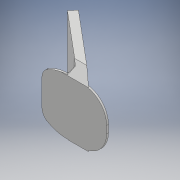
# Autodesk Inventor part: forJ
Saved by Autodesk Inventor 2018 (Build 220112000, 112)
## iProperties
Created: 2019-10-10
Part Number: forJ
Material: Типовые
Document SubType Name: Modeling
Designer: Professional
Density: 1 g/cm^3
Appearance: По умолчанию
Author: Professional
Autodesk Inventor part; units mm, degrees
ref_plane "YZ Plane" through (0, 0, 0) normal (1, 0, 0) x (0, 1, 0)
ref_plane "XZ Plane" through (0, 0, 0) normal (0, 1, 0) x (-1, 0, 0)
ref_plane "XY Plane" through (0, 0, 0) normal (0, 0, 1) x (1, 0, 0)
sketch "Эскиз1" plane through (0, 0, 0) normal (0, 1, 0) x (-1, 0, 0)
  arc A0 (-35, 4.9788) -> (-22, -8.0212) centre (-22, 4.9788) ccw
  line L0 (-22, -8.0212) -> (-13.0639, -8.0212)
  spline S0 degree 3 poles (-2.5479, -4.9591) (-3.2993, -5.4016) (-4.1343, -5.8409) (-5.9302, -6.6434) (-6.8964, -6.9949) (-8.5997, -7.4884) (-9.4965, -7.6913) (-11.3101, -7.9579) (-12.2269, -8.0212) (-13.0639, -8.0212) knots 10.698377 10.698377 10.698377 10.698377 10.956011 10.956011 11.236917 11.236917 11.488014 11.488014 11.739111 11.739111 11.739111 11.739111
  spline S1 degree 3 poles (0, 0) (0, -0.5347) (-0.0651, -1.0722) (-0.3672, -2.2857) (-0.6556, -2.9523) (-1.2591, -3.8313) (-1.4871, -4.1028) (-1.987, -4.5799) (-2.2566, -4.7875) (-2.5479, -4.9591) knots 0 0 0 0 0.160414 0.160414 0.374819 0.374819 0.480856 0.480856 0.582641 0.582641 0.582641 0.582641
  line L1 (0, 0) -> (0, 13.9576)
  spline S2 degree 3 poles (-2.5479, 18.9167) (-2.0742, 18.6377) (-1.6582, 18.264) (-0.8827, 17.3065) (-0.5589, 16.6952) (-0.114, 15.3778) (0, 14.665) (0, 13.9576) knots 0 0 0 0 0.164934 0.164934 0.368054 0.368054 0.578929 0.578929 0.578929 0.578929
  spline S3 degree 3 poles (-13.0639, 21.9788) (-12.2269, 21.9788) (-11.3101, 21.9155) (-9.4965, 21.6489) (-8.5997, 21.446) (-6.8964, 20.9525) (-5.9302, 20.601) (-4.1343, 19.7985) (-3.2993, 19.3592) (-2.5479, 18.9167) knots 16.305621 16.305621 16.305621 16.305621 16.556719 16.556719 16.807816 16.807816 17.088722 17.088722 17.346355 17.346355 17.346355 17.346355
  line L2 (-22, 21.9788) -> (-13.0639, 21.9788)
  arc A1 (-22, 21.9788) -> (-35, 8.9788) centre (-22, 8.9788) ccw
  line L3 (-35, 4.9788) -> (-35, 8.9788)
  line L4 (0, -8.0212) -> (-35, -8.0212)
  line L5 (-35, -8.0212) -> (-35, 21.9788)
  line L6 (-35, 21.9788) -> (0, 21.9788)
  line L7 (0, 21.9788) -> (0, -8.0212)
  point P0 (0, 0)
  point P1 (-27, -8.0212)
  dimension "d0" = 30
  dimension "d1" = 35
  dimension "d6" = 8.0212
  dimension "d7" = 35
  dimension "d8" = 0
  dimension "d10" = 0
  dimension "d11" = 0
  dimension "d12" = 0
  dimension "d13" = 0
  constraints: 16 end point, 4 point on circle, 2 centre point, 2 parallel, 1 horizontal, 1 perpendicular, 9 other
  measures "d0" distance between parallel lines of L2 L0
  measures "d1" distance between parallel lines of L1 L3
  measures "d6" distance from line of point (0, 0) L0
  measures "d7" distance from line of point (0, 0) L3
  measures "d8" distance between parallel lines of L0 L4
  measures "d10" distance from line of L1.start L7
  measures "d11" distance from line of point (0, 0) L7
  measures "d12" distance between parallel lines of L2 L6
  measures "d13" distance between parallel lines of L3 L5
sketch "Эскиз3" plane through (0, 0, 0) normal (0, 0, 1) x (1, 0, 0)
  line L0 (-10.0776, 0) -> (17.5, 0)
  line L1 (17.5, 0) -> (17.5, 23.1404)
  line L2 (17.5, 23.1404) -> (-10.0776, 23.1404)
  line L3 (-10.0776, 23.1404) -> (-10.0776, 0)
  line L4 (-10.0776, 23.1404) -> (17.5, 0)
  line L5 (-10.0776, 23.1404) -> (-8.792, 24.6724)
  line L6 (17.5, 0) -> (18.7856, 1.5321)
  line L7 (17.5, 0) -> (35, 0)
  line L8 (-8.792, 24.6724) -> (18.7856, 1.5321)
  point P0 (0, 0)
  dimension "d4" = 36
  dimension "d14" = 35
  dimension "d15" = 17.5
  dimension "d16" = 40
  dimension "d17" = 2
  dimension "d18" = 2
  constraints: 18 end point, 3 perpendicular, 2 horizontal, 2 parallel
  measures "d4" distance between parallel lines of L6 L5
  measures "d14" distance of point (0, 0) L7.end
  measures "d15" distance of L0.end point (0, 0)
  measures "d16" angle of L0 L4
  measures "d17" distance from line of L5.end L4
  measures "d18" distance from line of L6.end L4
extrude "Выдавливание2" add sketch "Эскиз3" along normal blind 24.75 and the other way blind 11.25 contours L4 L2 L8 L1 | L1 L8 L6 | L5 L8 L2
extrude "Выдавливание3" add sketch "Эскиз1" against normal blind 1 contours L3 A1 L2 S3 S2 L1 S1 S0 L0 A0
sketch "Эскиз4" plane through (-8.792, 24.6724, 24.75) normal (0.6427876, 0.7660444, 0) x (0.7660444, -0.6427876, 0)
  line L0 (36, -2) -> (-2, -2)
  line L1 (-2, -2) -> (-2, 38)
  line L2 (-2, 38) -> (36, 38)
  line L3 (36, 38) -> (36, -2)
  line L4 (36, 0) -> (0, 0) projected
  line L5 (0, 36) -> (0, 0) projected
  line L6 (0, 36) -> (36, 36) projected
  line L7 (0, 36) -> (0, 0) projected
  line L8 (0, 0) -> (36, 0)
  line L9 (36, 0) -> (36, 36)
  line L10 (36, 36) -> (0, 36)
  line L11 (0, 36) -> (0, 0)
  point P0 (22.5942, 24.75)
  dimension "d25" = 2
  dimension "d26" = 2
  dimension "d27" = 2
  constraints: 16 end point, 4 parallel, 2 horizontal, 2 perpendicular
  measures "d25" distance between parallel lines of L0 L4
  measures "d26" distance between parallel lines of L5 L1
  measures "d27" distance between parallel lines of L6 L2
extrude "Выдавливание4" add sketch "Эскиз4" along normal blind 2.2 and the other way blind 2 contours L0 L1 L2 L3 L6 L5 L4
sketch "Эскиз7" plane through (17.5, 0, 21.9788) normal (0.7660444, -0.6427876, 0) x (0, 0, -1)
  line L0 (-4.7712, 0) -> (0, 0) projected
  line L1 (35.2288, 4.2) -> (-4.7712, 4.2) projected
  line L2 (-4.7712, 0) -> (35.2288, 0)
  line L3 (35.2288, 0) -> (35.2288, 4.2)
  line L4 (35.2288, 4.2) -> (-4.7712, 4.2)
  line L5 (-4.7712, 4.2) -> (-4.7712, 0)
  point P0 (21.9788, -11.2488)
  constraints: 8 end point, 2 parallel, 1 horizontal, 1 perpendicular
extrude "Выдавливание7" add sketch "Эскиз7" along normal blind 10
sketch "Эскиз8" plane through (0, -1, 0) normal (0, -1, 0) x (1, 0, 0)
  line L0 (48.9689, -23.074) -> (-18.8787, -23.074)
  line L1 (-18.8787, -23.074) -> (-18.8787, 28.9329)
  line L2 (-18.8787, 28.9329) -> (48.9689, 28.9329)
  line L3 (48.9689, 28.9329) -> (48.9689, -23.074)
  point P0 (0, 0)
  constraints: 8 end point, 2 parallel, 1 horizontal, 1 perpendicular
extrude "Выдавливание8" cut sketch "Эскиз8" along normal blind 10
fillet "Сопряжение2" radius 3 4 edges at (-8.085, 25.5151, 24.75) (-8.085, 25.5151, -11.25) (19.4926, 2.3747, 24.75) (19.4926, 2.3747, -11.25)
chamfer "Фаска2" distance 3 angle 45 2 edges at (18.0959, -0.5, 21.9788) (18.0959, -0.5, -8.0212)
chamfer "Фаска3" distance 5 angle 45 2 edges at (21.9588, -1, 26.75) (21.9588, -1, -13.25)
sketch "Эскиз9" plane through (0, 0, 0) normal (0, 1, 0) x (1, 0, 0)
  line L0 (24.034, 7.8611) -> (24.034, -21.8187) projected
  line L1 (24.034, -6) -> (0, -6)
  line L2 (0, -6) -> (0, -8)
  line L3 (0, -8) -> (24.034, -8)
  line L4 (24.034, -8) -> (24.034, -6)
  point P0 (0, 0)
  dimension "d57" = 2
  dimension "d58" = 6
  constraints: 8 end point, 2 parallel, 1 horizontal, 1 perpendicular, 1 point on line
  measures "d57" distance between parallel lines of L3 L1
  measures "d58" distance from line of point (0, 0) L1
extrude "Выдавливание9" add sketch "Эскиз9" along normal blind 19.5
sketch "Эскиз10" plane through (-8.792, 24.6724, 21.75) normal (0.6427876, 0.7660444, 0) x (0.7660444, -0.6427876, 0)
  line L0 (36, 30) -> (36, 15.75) projected
  line L1 (6.6522, 9.9175) -> (36, 9.9175)
  line L2 (36, 9.9175) -> (36, 17.4595)
  line L3 (36, 17.4595) -> (6.6522, 17.4595)
  line L4 (6.6522, 17.4595) -> (6.6522, 9.9175)
  point P0 (22.5942, 21.75)
  constraints: 8 end point, 2 parallel, 1 horizontal, 1 perpendicular, 1 point on line
extrude "Выдавливание10" cut sketch "Эскиз10" along normal blind 19.5
sketch "Эскиз11" plane through (-7.3779, 26.3577, 24.75) normal (0.6427876, 0.7660444, 0) x (0.7660444, -0.6427876, 0)
  line L0 (41.0054, 16.75) -> (41.0054, 2.9313) projected
  line L1 (36, 33) -> (36, 3) projected
  line L2 (41.0054, 12.6702) -> (36, 12.6702)
  line L3 (36, 12.6702) -> (36, 23.7333)
  line L4 (36, 23.7333) -> (41.0054, 23.7333)
  line L5 (41.0054, 23.7333) -> (41.0054, 12.6702)
  point P0 (22.5942, 24.75)
  constraints: 8 end point, 2 parallel, 2 point on line, 1 horizontal, 1 perpendicular
extrude "Выдавливание11" cut sketch "Эскиз11" along normal blind 19.5
chamfer "Фаска4" distance 4 angle 45 2 edges at (17.5, 0, -1.625) (17.5, 0, 15.375)
